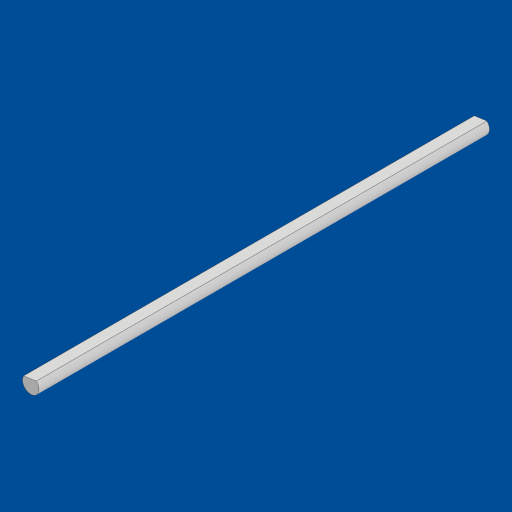
# Autodesk Inventor part: rod
Saved by Autodesk Inventor 2023.1 (Build 271208000, 208)
## iProperties
Created: 2023-06-05
Part Number: rod
Material: Generic
Document SubType Name: Modeling
Designer: nara atthama
Density: 1 g/cm^3
Appearance: Default
Author: nara atthama
Autodesk Inventor part; units mm, degrees
ref_plane "YZ Plane" through (0, 0, 0) normal (1, 0, 0) x (0, 1, 0)
ref_plane "XZ Plane" through (0, 0, 0) normal (0, 1, 0) x (-1, 0, 0)
ref_plane "XY Plane" through (0, 0, 0) normal (0, 0, 1) x (1, 0, 0)
sketch "Sketch1" plane through (0, 0, 0) normal (0, 0, 1) x (1, 0, 0)
  arc A0 (-1.3897, 0.8423) -> (1.1084, 1.1883) centre (0, 0) ccw
  line L0 (1.1084, 1.1883) -> (-1.3897, 0.8423)
  point P0 (-0.1407, 1.0153)
  dimension "d0" = 3.25
  dimension "d1" = 1.025
  constraints: 2 end point, 2 point on circle, 1 centre point, 1 coincident, 1 midpoint
  measures "d0" diameter of A0
  measures "d1" distance of point (0, 0) point (-0.141, 1.015)
extrude "Extrusion1" add sketch "Sketch1" along normal blind 89.6
body "Solid1"
